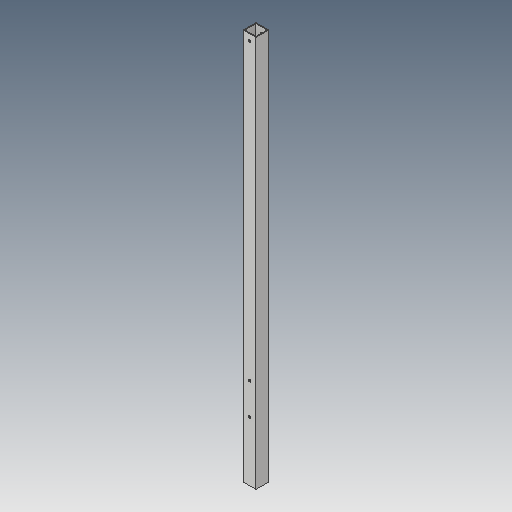
# Autodesk Inventor part: BaseSupportSQpipe
Saved by Autodesk Inventor 2019.4 (Build 234330000, 330)
## iProperties
Created: 2019-07-02
Part Number: BaseSupportSQpipe
Material: Generic
Document SubType Name: Modeling
Designer: AzLIer
Density: 1 g/cm^3
Appearance: Default
Author: AzLIer
Autodesk Inventor part; units mm, degrees
ref_plane "YZ Plane" through (0, 0, 0) normal (1, 0, 0) x (0, 1, 0)
ref_plane "XZ Plane" through (0, 0, 0) normal (0, 1, 0) x (-1, 0, 0)
ref_plane "XY Plane" through (0, 0, 0) normal (0, 0, 1) x (1, 0, 0)
sketch "スケッチ1" plane through (0, 0, 0) normal (0, 1, 0) x (-1, 0, 0)
  line L0 (-7.5, -7.5) -> (7.5, -7.5)
  line L1 (7.5, -7.5) -> (7.5, 7.5)
  line L2 (7.5, 7.5) -> (-7.5, 7.5)
  line L3 (-7.5, 7.5) -> (-7.5, -7.5)
  line L4 (-7.5, -7.5) -> (7.5, 7.5) construction
  line L5 (7.5, -7.5) -> (-7.5, 7.5) construction
  point P0 (0, 0)
  dimension "d0" = 15
  constraints: 12 end point, 2 midpoint, 2 parallel, 2 perpendicular, 1 horizontal
  measures "d0" distance of L2.end L1.end
extrude "押し出し1" add sketch "スケッチ1" along normal blind 460
shell "シェル1" thickness 1 removed faces 2 at (2.5, 0, 2.5) at (2.5, 460, 2.5)
sketch "スケッチ2" plane through (7.5, 0, -7.5) normal (0, 0, -1) x (-1, 0, 0)
  line L0 (7.5, 0) -> (7.5, 70) construction
  line L1 (0, 460) -> (15, 460) projected
  point P0 (7.5, 107)
  point P1 (7.5, 452.5)
  dimension "d4" = 37
  dimension "d5" = 70
  dimension "d13" = 7.5
  constraints: 2 end point, 2 point on line, 1 coincident, 1 vertical
  measures "d4" distance of point (7.5, 70) point (7.5, 107)
  measures "d5" distance of L0.start L0.end
  measures "d13" distance from line of L1 point (7.5, 452.5)
hole "穴1" at (0, 70, -7.5) at (0, 107, -7.5) at (0, 452.5, -7.5) direction (0, 0, 1) diameter 3.2 end through all
